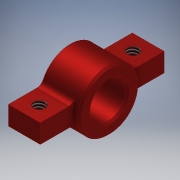
# Autodesk Inventor part: EPS_RBFPinHolder
Saved by Autodesk Inventor 2018 (Build 220112000, 112)
## iProperties
Created: 2018-05-29
Part Number: EPS_RBFPinHolder
Material: Aluminum 6061
Document SubType Name: Modeling
Designer: Bradley
Density: 2.7 g/cm^3
Appearance: Anodized - Red
Author: Bradley
Autodesk Inventor part; units mm, degrees
ref_plane "YZ Plane" through (0, 0, 0) normal (1, 0, 0) x (0, 1, 0)
ref_plane "XZ Plane" through (0, 0, 0) normal (0, 1, 0) x (-1, 0, 0)
ref_plane "XY Plane" through (0, 0, 0) normal (0, 0, 1) x (1, 0, 0)
sketch "Sketch1" plane through (0, 0, 0) normal (1, 0, 0) x (0, 1, 0)
  circle A0 centre (0, 0) radius 2.3812 construction
  circle A1 centre (0, 0) radius 2.425
  line L0 (-8.2653, 1.15) -> (-8.2653, -1.35)
  line L1 (-8.2653, -1.35) -> (-4.4133, -1.35)
  line L2 (-8.2653, 1.15) -> (-4.5141, 1.15)
  arc A2 (3.6113, 1.72) -> (-3.6113, 1.72) centre (0, 0) ccw
  arc A3 (-3.5307, -1.88) -> (3.5307, -1.88) centre (0, 0) ccw
  line L3 (4.5141, 1.15) -> (8.2653, 1.15)
  line L4 (8.2653, 1.15) -> (8.2653, -1.35)
  line L5 (8.2653, -1.35) -> (4.4133, -1.35)
  arc A4 (-4.5141, 1.15) -> (-3.6113, 1.72) centre (-4.5141, 2.15) ccw
  arc A5 (-3.5307, -1.88) -> (-4.4133, -1.35) centre (-4.4133, -2.35) ccw
  arc A6 (4.4133, -1.35) -> (3.5307, -1.88) centre (4.4133, -2.35) ccw
  arc A7 (3.6113, 1.72) -> (4.5141, 1.15) centre (4.5141, 2.15) ccw
  point P0 (-3.7653, -1.35)
  point P1 (-3.8311, 1.15)
  point P2 (3.8311, 1.15)
  point P3 (3.7653, -1.35)
  dimension "d0" = 4.7625
  dimension "d1" = 4.85
  dimension "d2" = 0.0437
  dimension "d3" = 4
  dimension "d4" = 1.575
  dimension "d5" = 1.35
  dimension "d6" = 2.5
  dimension "d7" = 4.5
  dimension "d8" = 16.5306
  dimension "d9" = 1
  constraints: 17 point on circle, 12 end point, 8 centre point, 8 tangent, 4 point on line, 3 equal radius, 3 perpendicular, 2 coincident, 2 concentric, 2 equal length, 2 horizontal, 1 collinear, 1 vertical
  measures "d0" diameter of A0
  measures "d1" diameter of A1
  measures "d2" radial gap between concentric circles of A0 A1
  measures "d3" radius of A2
  measures "d4" radial gap between concentric circles of A1 A2
  measures "d5" distance from line of point (0, 0) L1
  measures "d6" distance of L0.start L0.end
  measures "d7" distance of L0.end point (-3.765, -1.35)
  measures "d8" distance between parallel lines of L4 L0
  measures "d9" radius of A4
extrude "Extrusion1" add sketch "Sketch1" along normal mid plane 4.25
sketch "Sketch2" plane through (2.125, 0, 0) normal (1, 0, 0) x (0, 0, -1)
  circle A0 centre (0, 0) radius 2.425 projected
  line L0 (-1.15, -8.2653) -> (1.35, -8.2653) projected
  line L1 (1.35, -8.2653) -> (1.35, -4.4133) projected
  arc A1 (1.88, -3.5307) -> (1.35, -4.4133) centre (2.35, -4.4133) ccw projected
  arc A2 (1.88, -3.5307) -> (1.88, 3.5307) centre (0, 0) ccw projected
  arc A3 (1.35, 4.4133) -> (1.88, 3.5307) centre (2.35, 4.4133) ccw projected
  line L2 (1.35, 4.4133) -> (1.35, 8.2653) projected
  line L3 (1.35, 8.2653) -> (-1.15, 8.2653) projected
  line L4 (-1.15, 8.2653) -> (-1.15, 4.5141) projected
  arc A4 (-1.72, 3.6113) -> (-1.15, 4.5141) centre (-2.15, 4.5141) ccw projected
  arc A5 (-1.72, 3.6113) -> (-1.72, -3.6113) centre (0, 0) ccw projected
  arc A6 (-1.15, -4.5141) -> (-1.72, -3.6113) centre (-2.15, -4.5141) ccw projected
  line L5 (-1.15, -4.5141) -> (-1.15, -8.2653) projected
  arc A7 (-1.72, 3.6113) -> (-1.72, -3.6113) centre (0, 0) ccw projected
  circle A8 centre (0, 0) radius 4
  constraints: 1 coincident, 3 other
extrude "Extrusion2" add sketch "Sketch2" along normal blind 1 contours A5 A8 A2
chamfer "Chamfer1" distance 0.25 angle 45 3 edges at (3.125, 0, 4) (3.125, 0, 2.425) (-2.125, -2.425, 0)
sketch "Sketch3" plane through (2.125, -4.4133, -1.35) normal (0, 0, -1) x (-1, 0, 0)
  line L0 (4.25, 0) -> (0, 0) projected
  line L1 (0, -3.852) -> (0, 0) projected
  line L2 (4.25, -3.852) -> (0, -3.852) projected
  line L3 (4.25, 0) -> (4.25, -3.852) projected
  line L4 (4.25, 12.6786) -> (0, 12.6786) projected
  line L5 (0, 8.8267) -> (0, 12.6786) projected
  line L6 (4.25, 8.8267) -> (0, 8.8267) projected
  line L7 (4.25, 12.6786) -> (4.25, 8.8267) projected
  line L8 (2.125, -1.8367) -> (2.125, 10.6633) construction
  line L9 (4.25, 0.8827) -> (4.25, 7.944) projected
  point P0 (2.125, 4.4133)
  point P1 (4.25, 4.4133)
  point P2 (2.125, -3.852)
  point P3 (2.125, 4.4133)
  dimension "d17" = 12.5
  constraints: 3 coincident, 3 midpoint, 2 end point, 1 horizontal alignment, 1 vertical, 1 vertical alignment
  measures "d17" distance of L8.start L8.end
hole "Hole1" at (0, -6.25, -1.35) at (0, 6.25, -1.35) direction (0, 0, 1) diameter 1.567 end through all thread size "M2x0.4" class "6H" standard "ANSI Metric M Profile"
body "Solid1"
